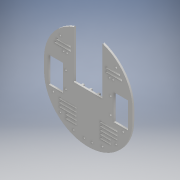
# Autodesk Inventor part: LBase
Saved by Autodesk Inventor 2017 (Build 210142000, 142)
## iProperties
Part Number: LBase
Material: Genérico
Document SubType Name: Modeling
Designer: Roberto
Density: 1 g/cm^3
Appearance: Valor por defecto
Author: Roberto
Autodesk Inventor part; units mm, degrees
ref_plane "YZ Plane" through (0, 0, 0) normal (1, 0, 0) x (0, 1, 0)
ref_plane "XZ Plane" through (0, 0, 0) normal (0, 1, 0) x (-1, 0, 0)
ref_plane "XY Plane" through (0, 0, 0) normal (0, 0, 1) x (1, 0, 0)
sketch "Boceto1" plane through (0, 0, 0) normal (0, 1, 0) x (-1, 0, 0)
  circle A0 centre (1.848, -3.409) radius 0.15
  circle A1 centre (-6.552, -3.409) radius 0.15
  circle A2 centre (-5.952, -3.409) radius 0.15
  circle A3 centre (1.248, -3.409) radius 0.15
  line L0 (2.573, -11.109) -> (2.573, -11.409)
  line L1 (2.573, -11.409) -> (-0.327, -11.409)
  line L2 (-0.327, -11.409) -> (-0.327, -11.109)
  line L3 (-0.327, -11.109) -> (2.573, -11.109)
  line L4 (-7.277, -12.009) -> (-7.277, -11.709)
  line L5 (-7.277, -11.709) -> (-4.377, -11.709)
  line L6 (-4.377, -11.709) -> (-4.377, -12.009)
  line L7 (-4.377, -12.009) -> (-7.277, -12.009)
  line L8 (-7.277, -10.509) -> (-4.377, -10.509)
  line L9 (-4.377, -10.509) -> (-4.377, -10.809)
  line L10 (-4.377, -10.809) -> (-7.277, -10.809)
  line L11 (-7.277, -10.809) -> (-7.277, -10.509)
  line L12 (0.648, -2.9395) -> (0.648, -2.6395)
  line L13 (0.648, -2.6395) -> (3.348, -2.6395)
  line L14 (3.348, -2.6395) -> (3.348, -2.9395)
  line L15 (3.348, -2.9395) -> (0.648, -2.9395)
  line L16 (0.648, -2.3395) -> (0.648, -2.0395)
  line L17 (0.648, -2.0395) -> (3.048, -2.0395)
  line L18 (3.048, -2.0395) -> (3.048, -2.3395)
  line L19 (3.048, -2.3395) -> (0.648, -2.3395)
  line L20 (-0.327, -12.309) -> (1.473, -12.309)
  line L21 (1.473, -12.309) -> (1.473, -12.609)
  line L22 (1.473, -12.609) -> (-0.327, -12.609)
  line L23 (-0.327, -12.609) -> (-0.327, -12.309)
  line L24 (-6.177, -12.609) -> (-6.177, -12.309)
  line L25 (-6.177, -12.309) -> (-4.377, -12.309)
  line L26 (-4.377, -12.309) -> (-4.377, -12.609)
  line L27 (-4.377, -12.609) -> (-6.177, -12.609)
  line L28 (-6.177, -13.209) -> (-6.177, -12.909)
  line L29 (-6.177, -12.909) -> (-4.377, -12.909)
  line L30 (-4.377, -12.909) -> (-4.377, -13.209)
  line L31 (-4.377, -13.209) -> (-6.177, -13.209)
  line L32 (-0.327, -13.209) -> (-0.327, -12.909)
  line L33 (-0.327, -12.909) -> (1.473, -12.909)
  line L34 (1.473, -12.909) -> (1.473, -13.209)
  line L35 (1.473, -13.209) -> (-0.327, -13.209)
  line L36 (-5.352, -2.0395) -> (-5.352, -2.3395)
  line L37 (-5.352, -2.3395) -> (-7.752, -2.3395)
  line L38 (-7.752, -2.3395) -> (-7.752, -2.0395)
  line L39 (-7.752, -2.0395) -> (-5.352, -2.0395)
  line L40 (-5.352, -2.6395) -> (-5.352, -2.9395)
  line L41 (-5.352, -2.9395) -> (-8.052, -2.9395)
  line L42 (-8.052, -2.9395) -> (-8.052, -2.6395)
  line L43 (-8.052, -2.6395) -> (-5.352, -2.6395)
  line L44 (-7.277, -11.409) -> (-7.277, -11.109)
  line L45 (-7.277, -11.109) -> (-4.377, -11.109)
  line L46 (-4.377, -11.109) -> (-4.377, -11.409)
  line L47 (-4.377, -11.409) -> (-7.277, -11.409)
  line L48 (-0.327, -12.009) -> (-0.327, -11.709)
  line L49 (-0.327, -11.709) -> (2.573, -11.709)
  line L50 (2.573, -11.709) -> (2.573, -12.009)
  line L51 (2.573, -12.009) -> (-0.327, -12.009)
  line L52 (2.573, -10.809) -> (-0.327, -10.809)
  line L53 (-0.327, -10.809) -> (-0.327, -10.509)
  line L54 (-0.327, -10.509) -> (2.573, -10.509)
  line L55 (2.573, -10.509) -> (2.573, -10.809)
  circle A4 centre (0.1196, -14.109) radius 0.15
  circle A5 centre (-4.752, -14.109) radius 0.15
  circle A6 centre (3.5677, -10.209) radius 0.15
  circle A7 centre (-8.2717, -10.209) radius 0.15
  line L56 (-4.752, 0.9966) -> (-4.752, -7.109)
  arc A8 (-4.752, 0.9966) -> (-9.852, -6.109) centre (-2.352, -6.109) ccw
  line L57 (-9.852, -7.909) -> (-9.852, -6.109)
  arc A9 (-9.852, -7.909) -> (5.148, -7.909) centre (-2.352, -7.909) ccw
  line L58 (5.148, -6.109) -> (5.148, -7.909)
  arc A10 (5.148, -6.109) -> (0.048, 0.9966) centre (-2.352, -6.109) ccw
  line L59 (0.048, -7.109) -> (0.048, 0.9966)
  line L60 (-9.077, -9.609) -> (-9.077, -5.209)
  line L61 (-9.077, -5.209) -> (-6.677, -5.209)
  line L62 (-6.677, -5.209) -> (-6.677, -9.609)
  line L63 (-6.677, -9.609) -> (-9.077, -9.609)
  line L64 (1.948, -9.609) -> (1.948, -5.209)
  line L65 (1.948, -5.209) -> (4.348, -5.209)
  line L66 (4.348, -5.209) -> (4.348, -9.609)
  line L67 (4.348, -9.609) -> (1.948, -9.609)
  circle A11 centre (-7.086, -1.375) radius 0.15
  circle A12 centre (2.382, -1.375) radius 0.15
  circle A13 centre (-7.086, -12.643) radius 0.15
  circle A14 centre (2.382, -12.643) radius 0.15
  circle A15 centre (-6.152, -6.015) radius 0.15
  circle A16 centre (-6.152, -8.803) radius 0.15
  circle A17 centre (1.448, -6.015) radius 0.15
  circle A18 centre (1.448, -8.803) radius 0.15
  circle A19 centre (-1.677, -14.409) radius 0.15
  circle A20 centre (-3.027, -14.409) radius 0.15
  line L68 (0.048, -7.109) -> (-4.752, -7.109)
  line L69 (-0.852, -7.109) -> (0.048, -7.109)
  line L70 (-4.752, -7.109) -> (-3.852, -7.109)
  line L71 (-1.152, -12.909) -> (-1.152, -7.109)
  line L72 (-2.202, -7.109) -> (-1.152, -7.109)
  line L73 (-2.202, -7.109) -> (-2.202, -12.909)
  line L74 (-2.202, -12.909) -> (-2.502, -12.909)
  line L75 (-2.502, -12.909) -> (-2.502, -7.109)
  line L76 (-3.552, -7.109) -> (-2.502, -7.109)
  line L77 (-3.552, -7.109) -> (-3.552, -12.909)
  line L78 (-3.852, -12.909) -> (-3.852, -7.109)
  line L79 (-0.852, -7.109) -> (-0.852, -12.909)
  line L80 (-0.852, -12.909) -> (-1.152, -12.909)
  line L81 (-3.552, -12.909) -> (-3.852, -12.909)
  point P0 (0, 0)
  point P1 (0, 0.8)
  point P2 (-2.352, -7.109)
  constraints: 164 end point, 21 centre point, 6 point on circle, 1 horizontal
extrude "Extrusión1" add sketch "Boceto1" along normal blind 0.3
sketch "Boceto2" plane through (0, 0.3, 0) normal (0, 1, 0) x (1, 0, 0)
  line L0 (-9.852, -7.909) -> (-9.852, -6.109)
  line L1 (-0.048, 7.109) -> (4.752, 7.109) projected
  line L2 (1.152, 7.109) -> (2.202, 7.109)
  line L3 (3.852, 7.109) -> (4.752, 7.109)
  line L4 (2.502, 7.109) -> (3.552, 7.109)
  line L5 (-0.048, 7.109) -> (0.852, 7.109)
  line L6 (4.752, 7.109) -> (-0.048, 7.109)
  line L7 (3.852, 12.909) -> (3.552, 12.909)
  line L8 (2.502, 12.909) -> (2.202, 12.909)
  line L9 (0.852, 12.909) -> (0.852, 7.109)
  line L10 (1.152, 7.109) -> (1.152, 12.909)
  line L11 (2.202, 12.909) -> (2.202, 7.109)
  line L12 (2.502, 7.109) -> (2.502, 12.909)
  line L13 (3.552, 12.909) -> (3.552, 7.109)
  line L14 (3.852, 7.109) -> (3.852, 12.909)
  line L15 (1.152, 12.909) -> (0.852, 12.909)
  line L16 (0.852, 7.109) -> (1.152, 7.109)
  line L17 (1.152, 7.109) -> (1.152, 12.909)
  line L18 (1.152, 12.909) -> (0.852, 12.909)
  line L19 (0.852, 12.909) -> (0.852, 7.109)
  line L20 (2.202, 12.909) -> (2.502, 12.909)
  line L21 (2.502, 12.909) -> (2.502, 7.109)
  line L22 (2.502, 7.109) -> (2.202, 7.109)
  line L23 (2.202, 7.109) -> (2.202, 12.909)
  line L24 (3.552, 12.909) -> (3.852, 12.909)
  line L25 (3.852, 12.909) -> (3.852, 7.109)
  line L26 (3.852, 7.109) -> (3.552, 7.109)
  line L27 (3.552, 7.109) -> (3.552, 12.909)
  point P0 (2.352, 7.109)
  point P1 (2.352, 7.909)
  constraints: 54 end point, 6 parallel, 4 horizontal, 3 perpendicular
sketch "Boceto3" plane through (-0.048, 0, -7.109) normal (0, 0, 1) x (1, 0, 0)
  line L0 (0, 0) -> (4.8, 0)
  line L1 (4.8, 0) -> (4.8, 0.3)
  line L2 (0, 0.3) -> (4.8, 0.3)
  line L3 (0, 0) -> (0, 0.3)
  line L4 (-0.15, 0.15) -> (0, 0)
  line L5 (-0.15, 0.15) -> (0, 0.3)
  line L6 (0, 0.3) -> (4.8, 0.3)
  line L7 (9.9, 0.3) -> (-5.1, 0.3)
  line L8 (4.8, 0.3) -> (4.8, 0)
  line L9 (4.95, 0.15) -> (4.8, 0.3)
  line L10 (4.95, 0.15) -> (4.8, 0)
  line L11 (4.8, 0) -> (0, 0)
  line L12 (9.9, 0) -> (-5.1, 0)
  point P0 (0.048, 0)
  point P1 (4.752, 0)
  constraints: 26 end point, 2 collinear, 1 perpendicular
extrude "Extrusión2" cut sketch "Boceto3" along normal blind 12
extrude "Extrusión3" add sketch "Boceto2" along normal blind 0.3
